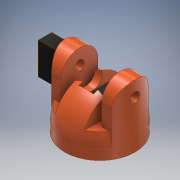
# Autodesk Inventor part: base_m1
Saved by Autodesk Inventor 2017 (Build 210142000, 142)
## iProperties
Created: 2017-02-24
Part Number: base_m1
Material: Phenolic Resin
Document SubType Name: Modeling
Designer: Canton
Density: 1.38 g/cm^3
Appearance: Smooth - Light Orange
Author: Canton
Autodesk Inventor part; units mm, degrees
sketch "Sketch1" plane through (0, 0, 0) normal (0, 0, 1) x (1, 0, 0)
  circle A0 centre (0, 0) radius 53.5
  dimension "d0" = 107
  constraints: 1 centre point, 1 coincident
  measures "d0" diameter of A0
extrude "Extrusion1" add sketch "Sketch1" along normal blind 18
ref_plane "Work Plane1" through (0, 0, 0) normal (1, 0, 0) x (0, 1, 0)
sketch "Sketch2" plane through (0, 0, 0) normal (1, 0, 0) x (0, 1, 0)
  line L0 (53.5, 18) -> (-53.5, 18) projected
  arc A0 (53.5, 18) -> (0, 71.5) centre (0, 18) ccw
  line L1 (0, 18) -> (0, 71.5)
  line L2 (0, 18) -> (53.5, 18)
  point P0 (0, 0)
  constraints: 5 end point, 3 point on circle, 1 centre point, 1 midpoint, 1 perpendicular, 1 point on line
revolve "Revolution1" add sketch "Sketch2" angle 360 about axis through (0, 0, 18) along (0, 0, 1)
ref_plane "Work Plane3" through (0, 0, 36) normal (0, 0, 1) x (1, 0, 0)
ref_plane "Work Plane2" through (0, 0, 0) normal (0, 0, 1) x (1, 0, 0)
sketch "Sketch11" plane through (0, 0, 36) normal (0, 0, 1) x (1, 0, 0)
  line L0 (-22, 48.7673) -> (-22, -48.7673)
  line L1 (22, -48.7673) -> (22, 48.7673)
  arc A0 (22, -48.7673) -> (22, 48.7673) centre (0, 0) ccw
  arc A1 (-22, 48.7673) -> (-22, -48.7673) centre (0, 0) ccw
  constraints: 4 end point, 4 point on circle, 2 centre point, 1 coincident, 1 parallel
extrude "Extrusion5" cut sketch "Sketch11" along normal blind 60
sketch "Sketch12" plane through (0, 0, 36) normal (0, 0, 1) x (1, 0, 0)
  line L0 (-45.5878, 28) -> (-31, 28)
  line L1 (-45.5878, -28) -> (-31, -28)
  line L2 (-31, 28) -> (-31, -28)
  arc A0 (-45.5878, 28) -> (-45.5878, -28) centre (0, 0) ccw
  line L3 (45.5878, 28) -> (31, 28)
  line L4 (45.5878, -28) -> (31, -28)
  line L5 (31, 28) -> (31, -28)
  arc A1 (45.5878, -28) -> (45.5878, 28) centre (0, 0) ccw
  constraints: 12 end point, 4 point on circle, 2 centre point, 1 coincident
extrude "Extrusion6" cut sketch "Sketch12" against normal blind 18 contours L0 L2 L1 A0
extrude "Extrusion7" cut sketch "Sketch12" against normal blind 18 contours A1 L4 L5 L3
sketch "Sketch13" plane through (0, 0, 18) normal (0, 0, 1) x (1, 0, 0)
  arc A0 (-45.5878, 28) -> (-45.5878, -28) centre (0, 0) ccw
  line L0 (-31, 28) -> (-31, -28) projected
  line L1 (-31, 28) -> (-45.5878, 28)
  line L2 (-45.5878, -28) -> (-31, -28)
  line L3 (-31, -28) -> (-31, 28)
  constraints: 6 end point, 2 point on circle, 1 centre point, 1 coincident, 1 horizontal, 1 parallel
extrude "Extrusion8" add sketch "Sketch13" along normal blind 77.5
ref_plane "Work Plane4" through (-31, 0, 95.5) normal (1, 0, 0) x (0, 0, -1)
sketch "Sketch18" plane through (-31, 0, 95.5) normal (1, 0, 0) x (0, 0, -1)
  arc A0 (0, 0) -> (28, -28) centre (28, 0) ccw
  line L0 (0, 0) -> (0, -28)
  line L1 (0, -28) -> (28, -28)
  point P0 (95.5, 0)
  constraints: 4 end point, 2 point on circle, 1 centre point, 1 perpendicular, 1 tangent, 1 vertical
extrude "Extrusion9" cut sketch "Sketch18" against normal blind 22.5
sketch "Sketch19" plane through (-31, 0, 95.5) normal (1, 0, 0) x (0, 0, -1)
  arc A0 (28, 28) -> (0, 0) centre (28, 0) ccw
  line L0 (0, 28) -> (28, 28)
  line L1 (0, 0) -> (0, 28) projected
  line L2 (0, 28) -> (0, 0)
  point P0 (95.5, 0)
  constraints: 4 end point, 2 point on circle, 1 centre point, 1 vertical
extrude "Extrusion10" cut sketch "Sketch19" against normal blind 22.5
sketch "Sketch20" plane through (-31, 0, 95.5) normal (1, 0, 0) x (0, 0, -1)
  point P0 (95.5, 0)
ref_plane "Work Plane6" through (-53.5, 0, 0) normal (1, 0, 0) x (0, 1, 0)
sketch "Sketch21" plane through (-53.5, 0, 0) normal (1, 0, 0) x (0, 1, 0)
  circle A0 centre (0, 72.2) radius 7.5
  line L0 (-53.5, 0) -> (53.5, 0) projected
  dimension "d60" = 15
  dimension "d61" = 72.2
  constraints: 1 centre point
  measures "d60" diameter of A0
  measures "d61" distance from line of L0 A0.centre
extrude "Extrusion11" cut sketch "Sketch21" along normal blind 22.5
ref_plane "Work Plane7" through (22, 0, 66.7673) normal (1, 0, 0) x (0, 0, -1)
sketch "Sketch23" plane through (22, 0, 66.7673) normal (1, 0, 0) x (0, 0, -1)
  circle A0 centre (2.7673, 0) radius 15
  point P0 (66.7673, 0)
  constraints: 1 centre point
extrude "Extrusion12" cut sketch "Sketch23" against normal blind 44
ref_plane "Work Plane8" through (0, 0, 66.7673) normal (1, 0, 0) x (0, 0, -1)
mirror "Mirror1" about plane through (0, 0, 66.7673) normal (1, 0, 0) of "Extrusion11", "Extrusion8", "Extrusion9"
ref_plane "Work Plane9" through (31, 0, 95.5) normal (-1, 0, 0) x (0, 0, 1)
sketch "Sketch24" plane through (31, 0, 95.5) normal (-1, 0, 0) x (0, 0, 1)
  arc A0 (0, 0) -> (-28, 28) centre (-28, 0) ccw
  line L0 (0, 28) -> (-28, 28)
  line L1 (0, 28) -> (0, 0)
  point P0 (-95.5, 0)
  constraints: 4 end point, 2 point on circle, 1 centre point, 1 coincident
extrude "Extrusion13" cut sketch "Sketch24" against normal blind 22.5
sketch "Sketch27" plane through (0, 0, 36) normal (0, 0, 1) x (1, 0, 0)
  arc A0 (11.25, 49.1089) -> (-11.25, 49.1089) centre (0, 0) ccw
  line L0 (-11.25, 0) -> (-11.25, 49.1089)
  line L1 (11.25, 0) -> (11.25, 49.1089)
  line L2 (-11.25, 49.1089) -> (-11.25, -21.1282)
  line L3 (-11.25, -21.1282) -> (11.25, -21.1282)
  line L4 (11.25, -21.1282) -> (11.25, 49.1089)
  constraints: 10 end point, 2 point on circle, 1 centre point, 1 parallel, 1 point on line
extrude "Extrusion14" cut sketch "Sketch27" along normal blind 60
sketch "Sketch28" plane through (0, 0, 36) normal (0, 0, 1) x (1, 0, 0)
  line L0 (-10.5, -10.5641) -> (10.5, -10.5641)
  line L1 (10.5, -10.5641) -> (10.5, 38.4359)
  line L2 (10.5, 38.4359) -> (-10.5, 38.4359)
  line L3 (-10.5, 38.4359) -> (-10.5, -10.5641)
  constraints: 8 end point, 2 parallel, 1 horizontal, 1 perpendicular
extrude "Extrusion15" add sketch "Sketch28" along normal blind 13
ref_plane "Work Plane13" through (-53.5, 0, 95.5) normal (-1, 0, 0) x (0, -1, 0)
sketch "Sketch29" plane through (-53.5, 0, 95.5) normal (-1, 0, 0) x (0, -1, 0)
  line L0 (10.25, -11.0943) -> (10.25, -59.5)
  line L1 (10.25, -59.5) -> (-10.25, -59.5)
  line L2 (-10.25, -11.0943) -> (-10.25, -59.5)
  line L3 (-10.25, -11.0943) -> (10.25, -11.0943)
  point P0 (0, -95.5)
  constraints: 8 end point, 1 perpendicular
extrude "Extrusion16" add sketch "Sketch29" along normal blind 30
body "Solid1"
